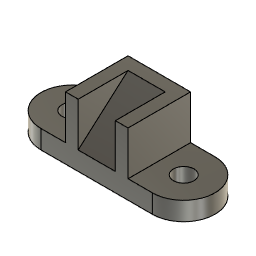
A2 (Autodesk Fusion 360 design; units mm, degrees)
Autodesk Fusion 360 part; units mm, degrees
sketch "Sketch1" plane through (0, 0, 0) normal (0, 0, 1) x (1, 0, 0)
  line L0 (0, 0) -> (-178, 0)
  line L1 (-178, 0) -> (-178, 64)
  line L2 (-178, 64) -> (0, 64)
  line L3 (0, 64) -> (0, 0)
  dimension "d1" = 64
  dimension "d2" = 178
  constraint horizontal L0
  constraint vertical L1
  constraint horizontal L2
  constraint vertical L3
  constraint coincident L0.start L3.end
  measures "d1" distance of L0.start L2.end
  measures "d2" distance of L0.start L0.end
extrude "Extrude1" add sketch "Sketch1" along normal blind 19
fillet "Fillet1" radius 32 4 edges at (0, 0, 9.5) (0, 64, 9.5) (-178, 0, 9.5) (-178, 64, 9.5)
sketch "Sketch2" plane through (0, 0, 19) normal (0, 0, 1) x (-1, 0, 0)
  arc A0 (146, -64) -> (146, 0) centre (146, -32) ccw
  line L0 (146, 0) -> (32, 0)
  arc A1 (32, 0) -> (32, -64) centre (32, -32) ccw
  line L1 (32, -64) -> (146, -64)
  line L2 (89, -64) -> (89, 0) construction
  circle A2 centre (32, -32) radius 10.5
  circle A3 centre (146, -32) radius 10.5
  dimension "d6" = 21
  constraint midpoint L0 L2.end
  constraint midpoint L1 L2.start
  constraint symmetric L2 A2 A3
  measures "d6" diameter of A2
extrude "Extrude2" cut sketch "Sketch2" against normal blind 90 contours A2 | A3
sketch "Sketch3" plane through (0, 0, 19) normal (0, 0, 1) x (-1, 0, 0)
  circle A0 centre (32, -32) radius 10.5
  circle A1 centre (146, -32) radius 10.5
  arc A2 (146, -64) -> (146, 0) centre (146, -32) ccw
  line L0 (146, 0) -> (32, 0)
  arc A3 (32, 0) -> (32, -64) centre (32, -32) ccw
  line L1 (32, -64) -> (146, -64)
  line L2 (146, -64) -> (32, -64) construction
  line L3 (89, -64) -> (89, 0) construction
  line L4 (89, -64) -> (57, -64)
  line L5 (121, -64) -> (108, -64)
  line L6 (108, -64) -> (108, 0)
  line L7 (108, 0) -> (121, 0)
  line L8 (121, 0) -> (121, -64)
  line L9 (121, -64) -> (108, -64)
  line L10 (108, -64) -> (108, 0)
  line L11 (108, 0) -> (121, 0)
  line L12 (121, 0) -> (121, -64)
  line L13 (70, -64) -> (70, 0)
  line L14 (57, -64) -> (70, -64)
  line L15 (57, 0) -> (57, -64)
  line L16 (70, 0) -> (57, 0)
  line L17 (108, -64) -> (70, -64)
  line L18 (70, -64) -> (70, -51)
  line L19 (70, -51) -> (108, -51)
  line L20 (108, -51) -> (108, -64)
  dimension "d9" = 32
  dimension "d10" = 32
  dimension "d11" = 13
  dimension "d12" = 64
  dimension "d13" = 13
  constraint coincident A2.start L1.end
  constraint coincident A3.end L1.start
  constraint midpoint L2 L3.start
  constraint midpoint L0 L3.end
  constraint perpendicular L3 L4
  constraint horizontal L5
  constraint vertical L6
  constraint horizontal L7
  constraint vertical L8
  constraint horizontal L9
  constraint vertical L10
  constraint horizontal L11
  constraint vertical L12
  constraint symmetric L3 L5.start L4.end
  constraint symmetric L3 L6.end L13.end
  constraint symmetric L3 L5.end L13.start
  constraint symmetric L3 L7.end L15.start
  constraint horizontal L17
  constraint vertical L18
  constraint horizontal L19
  constraint vertical L20
  constraint coincident L13 L18.end
  measures "d9" distance of L3.start L4.end
  measures "d10" distance of L3.start L5.start
  measures "d11" distance of L5.start L5.end
  measures "d12" distance of L5.start L7.end
  measures "d13" distance of L5.end L19.end
extrude "Extrude3" add sketch "Sketch3" along normal blind 45 contours L0 L1 L5 L6 L7 L8 L9 L10 L11 L12 L20 | L1 L4 L6 L10 L13 L17 L18 L19 L20 | L0 L1 L4 L13 L14 L15 L16 L18
sketch "Sketch4" plane through (-108, 0, 0) normal (1, 0, 0) x (0, 1, 0)
  line L0 (0, 19) -> (51, 19)
  line L1 (51, 19) -> (51, 64)
  line L2 (51, 64) -> (0, 64)
  line L3 (0, 64) -> (0, 19)
  line L4 (51, 64) -> (0, 19)
  line L5 (51, 19) -> (51, 64)
  line L6 (51, 19) -> (0, 19)
  constraint coincident L1.end L2.start
  constraint coincident L0.start L3.end
  constraint coincident L0.end L1.start
extrude "Extrude4" add sketch "Sketch4" along normal blind 38 contours L0 L1 L4 L5 L6
equation "d2 = 114 mm + 32 mm + 32 mm"
equation "d11 = ( ( 64 - 38 ) / 2 ) * 1 mm"
equation "d13 = 64 mm - 51 mm"
equation "d14 = 64 mm - 19 mm"
